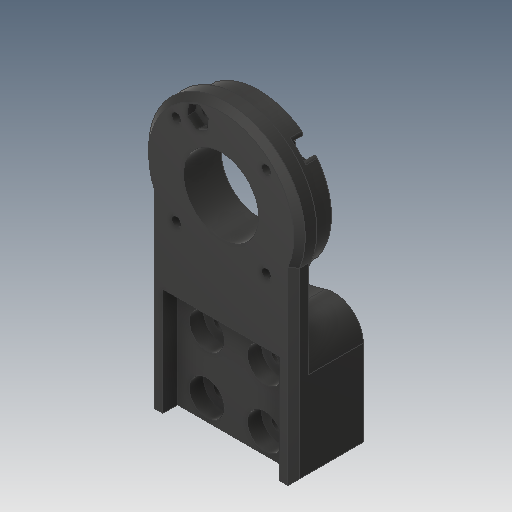
# Autodesk Inventor part: base_stepper
Saved by Autodesk Inventor 2020.3 (Build 243373000, 373)
## iProperties
Created: 2021-02-25
Part Number: base_stepper
Material: ABS Plastic
Document SubType Name: Modeling
Designer: paulg
Density: 1.06 g/cm^3
Appearance: Smooth - Black
Mass: 46.9238 g
Surface Area: 186.234 cm^2
Volume: 44.2678 cm^3
Author: paulg
Autodesk Inventor part; units mm, degrees
ref_plane "YZ Plane" through (0, 0, 0) normal (1, 0, 0) x (0, 1, 0)
ref_plane "XZ Plane" through (0, 0, 0) normal (0, 1, 0) x (-1, 0, 0)
ref_plane "XY Plane" through (0, 0, 0) normal (0, 0, 1) x (1, 0, 0)
sketch "Sketch1" plane through (0, 0, 0) normal (0, 0, 1) x (1, 0, 0)
  circle A0 centre (0, 0) radius 13
  circle A1 centre (0, 0) radius 25
  dimension "d0" = 50
  dimension "d1" = 26
  constraints: 2 centre point, 2 coincident
  measures "d0" diameter of A1
  measures "d1" diameter of A0
extrude "Extrusion1" add sketch "Sketch1" along normal blind 7
sketch "Sketch2" plane through (0, 0, 7) normal (0, 0, 1) x (1, 0, 0)
  circle A0 centre (0, 0) radius 13 projected
  circle A1 centre (0, 0) radius 25 projected
  circle A2 centre (0, 0) radius 27
  dimension "d4" = 2
  constraints: 1 centre point
  measures "d4" radial gap between concentric circles of A1 A2
extrude "Extrusion2" add sketch "Sketch2" along normal blind 1 contours A1 | A2
sketch "Sketch3" plane through (0, 0, 8) normal (0, 0, 1) x (1, 0, 0)
  circle A0 centre (0, 0) radius 13 projected
  circle A1 centre (0, 0) radius 27 projected
  line L0 (0, 0) -> (0, -42.599) construction
  circle A2 centre (0, 0) radius 27 projected
  line L1 (25, -75) -> (-25, -75)
  line L2 (-25, -75) -> (-25, -10.198)
  line L3 (-25, -10.198) -> (25, -10.198) construction
  line L4 (25, -10.198) -> (25, -75)
  line L5 (25, -75) -> (-25, -10.198) construction
  line L6 (-25, -75) -> (25, -10.198) construction
  arc A3 (-25, -10.198) -> (25, -10.198) centre (0, 0) ccw
  dimension "d7" = 50
  dimension "d8" = 75
  constraints: 14 end point, 2 midpoint, 2 parallel, 2 point on circle, 1 centre point, 1 coincident, 1 horizontal, 1 perpendicular, 1 vertical, 4 other
  measures "d7" distance of L1.start L1.end
  measures "d8" distance from line of L1 point (0, 0)
extrude "Extrusion3" add sketch "Sketch3" along normal blind 5
sketch "Sketch4" plane through (0, 0, 0) normal (0, 0, -1) x (-1, 0, 0)
  circle A0 centre (0, 0) radius 13 projected
  circle A1 centre (0, 0) radius 25 projected
  line L0 (15.5, -15.5) -> (-15.5, -15.5) construction
  line L1 (-15.5, -15.5) -> (-15.5, 15.5) construction
  line L2 (-15.5, 15.5) -> (15.5, 15.5) construction
  line L3 (15.5, 15.5) -> (15.5, -15.5) construction
  line L4 (15.5, -15.5) -> (-15.5, 15.5) construction
  line L5 (-15.5, -15.5) -> (15.5, 15.5) construction
  dimension "d11" = 31
  constraints: 12 end point, 4 coincident, 2 midpoint, 2 parallel, 2 perpendicular, 1 horizontal
  measures "d11" distance of L2.end L0.start
hole "Hole1" at (15.5, 15.5, 0) at (-15.5, 15.5, 0) at (-15.5, -15.5, 0) at (15.5, -15.5, 0) direction (0, 0, 1) diameter 3.2 end through all counterbore diameter 6.2 counterbore depth 4
fillet "Fillet1" radius 1 8 edges at (17.4081, 17.9432, 2) (17.9432, 17.4081, 2) (-17.4081, 17.9432, 2) (-17.9432, 17.4081, 2) (-17.9432, -17.4081, 2) (-17.4081, -17.9432, 2) (17.9432, -17.4081, 2) (17.4081, -17.9432, 2)
sketch "Sketch5" plane through (0, 0, 0) normal (0, 0, -1) x (-1, 0, 0)
  arc A0 (-14.4888, -18.4304) -> (-14.7527, -20.1831) centre (-14.1626, -19.3758) ccw projected
  arc A1 (-14.7527, -20.1831) -> (14.7527, -20.1831) centre (0, 0) ccw projected
  arc A2 (14.7527, -20.1831) -> (14.4888, -18.4304) centre (14.1626, -19.3758) ccw projected
  arc A3 (18.4304, -14.4888) -> (14.4888, -18.4304) centre (15.5, -15.5) ccw projected
  arc A4 (18.4304, -14.4888) -> (20.1831, -14.7527) centre (19.3758, -14.1626) ccw projected
  arc A5 (20.1831, -14.7527) -> (20.1831, 14.7527) centre (0, 0) ccw projected
  arc A6 (20.1831, 14.7527) -> (18.4304, 14.4888) centre (19.3758, 14.1626) ccw projected
  arc A7 (14.4888, 18.4304) -> (18.4304, 14.4888) centre (15.5, 15.5) ccw projected
  arc A8 (14.4888, 18.4304) -> (14.7527, 20.1831) centre (14.1626, 19.3758) ccw projected
  arc A9 (14.7527, 20.1831) -> (-14.7527, 20.1831) centre (0, 0) ccw projected
  arc A10 (-14.7527, 20.1831) -> (-14.4888, 18.4304) centre (-14.1626, 19.3758) ccw projected
  arc A11 (-18.4304, 14.4888) -> (-14.4888, 18.4304) centre (-15.5, 15.5) ccw projected
  arc A12 (-18.4304, 14.4888) -> (-20.1831, 14.7527) centre (-19.3758, 14.1626) ccw projected
  arc A13 (-20.1831, 14.7527) -> (-20.1831, -14.7527) centre (0, 0) ccw projected
  arc A14 (-20.1831, -14.7527) -> (-18.4304, -14.4888) centre (-19.3758, -14.1626) ccw projected
  arc A15 (-14.4888, -18.4304) -> (-18.4304, -14.4888) centre (-15.5, -15.5) ccw projected
  circle A16 centre (0, 0) radius 13 projected
  line L0 (0, 0) -> (0, 21) construction
  circle A17 centre (0, 0) radius 21 construction
  line L1 (0, 0) -> (8.0364, 19.4015) construction
  point P0 (-8.0364, 19.4015)
  point P1 (-19.4015, 8.0364)
  point P2 (-19.4015, -8.0364)
  point P3 (-8.0364, -19.4015)
  point P4 (8.0364, -19.4015)
  point P5 (19.4015, -8.0364)
  point P6 (19.4015, 8.0364)
  dimension "d20" = 22.5
  dimension "d23" = 360
  dimension "d25" = 42
  constraints: 4 end point, 2 coincident, 2 point on circle, 1 centre point, 1 vertical, 9 other
  measures "d20" angle of L1 L0
  measures "d25" diameter of A17
hole "Hole2" at (-8.0364, 19.4015, 0) at (8.0364, 19.4015, 0) at (19.4015, 8.0364, 0) at (19.4015, -8.0364, 0) at (8.0364, -19.4015, 0) at (-8.0364, -19.4015, 0) at (-19.4015, -8.0364, 0) at (-19.4015, 8.0364, 0) direction (0, 0, 1) diameter 3.3 depth 6 tip angle 118
sketch "Sketch6" plane through (0, 0, 8) normal (0, 0, -1) x (-1, 0, 0)
  arc A0 (-25, -10.198) -> (25, -10.198) centre (0, 0) ccw projected
  line L0 (-25, -10.198) -> (-25, -75) projected
  line L1 (-25, -75) -> (25, -75) projected
  line L2 (25, -75) -> (25, -10.198) projected
  line L3 (-25, -10.198) -> (-25, -75) projected
  arc A1 (-25, -25.9037) -> (25, -25.9037) centre (0, 0) ccw
  dimension "d33" = 36
  constraints: 2 point on circle, 2 point on line, 1 centre point, 1 coincident
  measures "d33" radius of A1
extrude "Extrusion4" add sketch "Sketch6" along normal blind 19 contours A1 L2 L1 L0
fillet "Fillet2" radius 10 2 edges at (-25, -25.9037, -1.5) (25, -25.9037, -1.5)
sketch "Sketch8" plane through (0, 0, 13) normal (0, 0, 1) x (1, 0, 0)
  circle A0 centre (-15.5, -15.5) radius 1.6 projected
  circle A1 centre (15.5, 15.5) radius 1.6 projected
  circle A2 centre (-15.5, 15.5) radius 1.6 projected
  circle A3 centre (15.5, -15.5) radius 1.6 projected
  circle A4 centre (0, 0) radius 13 projected
  line L0 (-25, -75) -> (25, -75) projected
  line L1 (25, -75) -> (25, -10.198) projected
  arc A5 (25, -10.198) -> (-25, -10.198) centre (0, 0) ccw projected
  line L2 (-25, -10.198) -> (-25, -75) projected
  line L3 (-12.0901, -38) -> (-12.0901, -60) projected
  line L4 (-12.0901, -38) -> (12.0929, -38) projected
  line L5 (12.0929, -60) -> (12.0929, -38) projected
  line L6 (-12.0901, -60) -> (12.0929, -60) projected
  line L7 (0, 0) -> (0.0014, -60)
  line L8 (-12.0901, -60) -> (12.0929, -60) projected
  line L9 (10.0013, -48) -> (-9.9987, -48) construction
  line L10 (-9.9987, -48) -> (-9.9987, -68) construction
  line L11 (-9.9987, -68) -> (10.0013, -68) construction
  line L12 (10.0013, -68) -> (10.0013, -48) construction
  line L13 (10.0013, -48) -> (-9.9987, -68) construction
  line L14 (-9.9987, -48) -> (10.0013, -68) construction
  point P0 (0.0013, -58)
  dimension "d43" = 20
  dimension "d68" = 20
  dimension "d69" = 10
  constraints: 14 end point, 3 coincident, 3 midpoint, 2 parallel, 1 horizontal, 1 perpendicular, 1 point on line
  measures "d43" distance of L10.end L11.end
  measures "d68" distance of L10.end L9.end
  measures "d69" distance between parallel lines of L9 L4
chamfer "Chamfer2" distance 2 angle 45 2 edges at (25, -42.599, 13) (-25, -42.599, 13)
chamfer "Chamfer3" distance 2 angle 45 3 edges at (24.0809, -12.2111, 13) (0, 27, 13) (-24.0809, -12.2111, 13)
chamfer "Chamfer4" distance 2 angle 45 2 edges at (25, -75, 0) (-25, -75, 0)
sketch "Sketch9" plane through (0, 0, 13) normal (0, 0, 1) x (1, 0, 0)
  circle A0 centre (-19.4015, -8.0364) radius 1.65 projected
  circle A1 centre (8.0364, -19.4015) radius 1.65 projected
  circle A2 centre (19.4015, 8.0364) radius 1.65 projected
  circle A3 centre (-8.0364, 19.4015) radius 1.65 projected
  circle A4 centre (8.0364, 19.4015) radius 1.65 projected
  circle A5 centre (19.4015, -8.0364) radius 1.65 projected
  circle A6 centre (-8.0364, -19.4015) radius 1.65 projected
  circle A7 centre (-19.4015, 8.0364) radius 1.65 projected
  arc A8 (14.7527, -20.1831) -> (14.4888, -18.4304) centre (14.1626, -19.3758) ccw projected
  arc A9 (-14.7527, -20.1831) -> (14.7527, -20.1831) centre (0, 0) ccw projected
  arc A10 (-14.4888, -18.4304) -> (-14.7527, -20.1831) centre (-14.1626, -19.3758) ccw projected
  arc A11 (-14.4888, -18.4304) -> (-18.4304, -14.4888) centre (-15.5, -15.5) ccw projected
  arc A12 (-20.1831, -14.7527) -> (-18.4304, -14.4888) centre (-19.3758, -14.1626) ccw projected
  arc A13 (-20.1831, 14.7527) -> (-20.1831, -14.7527) centre (0, 0) ccw projected
  arc A14 (-18.4304, 14.4888) -> (-20.1831, 14.7527) centre (-19.3758, 14.1626) ccw projected
  arc A15 (-18.4304, 14.4888) -> (-14.4888, 18.4304) centre (-15.5, 15.5) ccw projected
  arc A16 (-14.7527, 20.1831) -> (-14.4888, 18.4304) centre (-14.1626, 19.3758) ccw projected
  arc A17 (14.7527, 20.1831) -> (-14.7527, 20.1831) centre (0, 0) ccw projected
  arc A18 (14.4888, 18.4304) -> (14.7527, 20.1831) centre (14.1626, 19.3758) ccw projected
  arc A19 (14.4888, 18.4304) -> (18.4304, 14.4888) centre (15.5, 15.5) ccw projected
  arc A20 (20.1831, 14.7527) -> (18.4304, 14.4888) centre (19.3758, 14.1626) ccw projected
  arc A21 (20.1831, -14.7527) -> (20.1831, 14.7527) centre (0, 0) ccw projected
  arc A22 (18.4304, -14.4888) -> (20.1831, -14.7527) centre (19.3758, -14.1626) ccw projected
  arc A23 (18.4304, -14.4888) -> (14.4888, -18.4304) centre (15.5, -15.5) ccw projected
  circle A24 centre (0, 0) radius 13 projected
  circle A25 centre (-8.0364, 19.4015) radius 1.65 projected
  line L0 (-11.7702, 17.8549) -> (-11.2427, 21.8618)
  line L1 (-11.2427, 21.8618) -> (-7.5088, 23.4083)
  line L2 (-7.5088, 23.4083) -> (-4.3025, 20.9481)
  line L3 (-4.3025, 20.9481) -> (-4.8301, 16.9412)
  line L4 (-4.8301, 16.9412) -> (-8.5639, 15.3946)
  line L5 (-8.5639, 15.3946) -> (-11.7702, 17.8549)
  line L6 (0, 0) -> (-8.0364, 19.4015)
  dimension "d65" = 7
  constraints: 14 end point, 1 coincident, 1 perpendicular, 13 other
  measures "d65" distance between parallel lines of L4 L1
extrude "Extrusion6" cut sketch "Sketch9" against normal blind 3 contours A3 | L0 L1 L2 L3 L4 L5
sketch "Sketch10" plane through (-23, -75, -11) normal (0, -1, 0) x (1, 0, 0)
  line L0 (2.9, 10.1) -> (43.1, 10.1)
  line L1 (43.1, 10.1) -> (43.1, -10.1)
  line L2 (43.1, -10.1) -> (2.9, -10.1)
  line L3 (2.9, -10.1) -> (2.9, 10.1)
  line L4 (34.7391, 0) -> (11.2609, 0) projected
  line L5 (2.9, 10.1) -> (43.1, -10.1) construction
  line L6 (43.1, 10.1) -> (2.9, -10.1) construction
  line L7 (3, 10.7071) -> (3.7071, 10)
  line L8 (3.7071, 10) -> (3, 9.2929)
  line L9 (3, 9.2929) -> (2.2929, 10)
  line L10 (2.2929, 10) -> (3, 10.7071)
  line L11 (2.4, 10.6) -> (3.4, 9.6) construction
  line L12 (3.4, 10.6) -> (2.4, 9.6) construction
  line L13 (43, 10.7071) -> (43.7071, 10)
  line L14 (43.7071, 10) -> (43, 9.2929)
  line L15 (43, 9.2929) -> (42.2929, 10)
  line L16 (42.2929, 10) -> (43, 10.7071)
  line L17 (2.9, 29.1) -> (43.1, 29.1)
  line L18 (43.1, 29.1) -> (43.1, 18.9)
  line L19 (43.1, 18.9) -> (2.9, 18.9)
  line L20 (2.9, 18.9) -> (2.9, 29.1)
  line L21 (0, 24) -> (46, 24) projected
  line L22 (2.9, 29.1) -> (43.1, 18.9) construction
  line L23 (43.1, 29.1) -> (2.9, 18.9) construction
  point P0 (23, 11)
  point P1 (23, 0)
  point P2 (3, 0)
  point P3 (43, 0)
  point P4 (42.3929, 10.1)
  point P5 (43.1, 9.3929)
  point P6 (2.9, 9.3929)
  point P7 (3.6071, 10.1)
  point P8 (23, 24)
  point P9 (3.7071, 10)
  point P10 (43.1, 24)
  point P11 (2.9, 24)
  dimension "d70" = 40.2
  dimension "d71" = 20.2
  dimension "d75" = 1
  dimension "d76" = 1
  dimension "d77" = 1
  dimension "d78" = 1
  dimension "d79" = 40.2
  dimension "d80" = 10.2
  constraints: 44 end point, 8 midpoint, 8 parallel, 4 perpendicular, 2 horizontal
  measures "d70" distance of L1.end L2.end
  measures "d71" distance of L0.end L1.end
  measures "d75" distance of L8.end L9.end
  measures "d76" distance of L7.end L8.end
  measures "d77" distance of L14.end L15.end
  measures "d78" distance of L14.start L14.end
  measures "d79" distance of L18.end L19.end
  measures "d80" distance of L17.end L18.end
sketch "Sketch11" plane through (0, 0, 13) normal (0, 0, 1) x (1, 0, 0)
  circle A0 centre (-9.9987, -68) radius 2.5 projected
  circle A1 centre (10.0013, -48) radius 2.5 projected
  line L0 (-9.9987, -68) -> (10.0013, -68) construction
  line L1 (10.0013, -68) -> (10.0013, -48) construction
  line L2 (10.0013, -48) -> (-9.9987, -48) construction
  line L3 (-9.9987, -48) -> (-9.9987, -68) construction
  line L4 (-9.9987, -58) -> (10.0013, -58) construction
  line L5 (0.0013, -58) -> (0.0013, -38) construction
  line L6 (0.0013, -38) -> (-9.9987, -38) construction
  line L7 (0.0013, -38) -> (10.0013, -38) construction
  point P0 (0, 0)
  dimension "d72" = 20
  constraints: 16 end point, 3 midpoint, 3 perpendicular, 2 horizontal, 2 parallel
  measures "d72" distance of L5.start L5.end
extrude "Extrusion8" cut sketch "Sketch10" against normal blind 37 contours L3 L9 L10 L7 L0 | L0 L7 L8 L9 L3 | L0 L16 L15 L14 L1 L2 L3 L9 L8 L7 | L16 L13 L14 L1 L0 | L0 L1 L14 L15 L16 | L21 L18 L19 L20
sketch "Sketch12" plane through (-20.1, -75, 7.9) normal (0, 0, 1) x (1, 0, 0)
  line L0 (10, 27.0276) -> (30, 27.0276)
  line L1 (30, 27.0276) -> (30, 7.0276)
  line L2 (30, 7.0276) -> (10, 7.0276)
  line L3 (10, 7.0276) -> (10, 27.0276)
  line L4 (10, 27.0276) -> (30, 7.0276) construction
  line L5 (30, 27.0276) -> (10, 7.0276) construction
  point P0 (20.1, 75)
  point P1 (20, 17.0276)
  dimension "d83" = 20
  dimension "d84" = 20
  constraints: 12 end point, 2 midpoint, 2 parallel, 1 horizontal, 1 perpendicular
  measures "d83" distance of L1.end L2.end
  measures "d84" distance of L0.end L1.end
hole "Hole4" at (-10.1, -47.9724, 7.9) at (9.9, -47.9724, 7.9) at (9.9, -67.9724, 7.9) at (-10.1, -67.9724, 7.9) direction (0, 0, -1) diameter 5.5 end through all counterbore diameter 12 counterbore depth 5
sketch "Sketch13" plane through (0, 0, 10) normal (0, 0, 1) x (1, 0, 0)
  circle A0 centre (-8.0364, 19.4015) radius 1.65 projected
  circle A1 centre (-8.0364, 19.4015) radius 1.65
  point P0 (0, 0)
  constraints: 1 centre point, 1 coincident
sketch "Sketch14" plane through (0, 0, 10) normal (0, 0, 1) x (1, 0, 0)
  circle A0 centre (-8.0364, 19.4015) radius 1.65 projected
  circle A1 centre (-8.0364, 19.4015) radius 1.7
  point P0 (0, 0)
  dimension "d92" = 3.4
  constraints: 1 centre point, 1 coincident
  measures "d92" diameter of A1
extrude "Extrusion9" cut sketch "Sketch14" against normal through all contours A0 | A1
body "Solid1"
